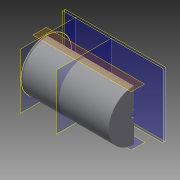
# Autodesk Inventor part: v1.0L
Saved by Autodesk Inventor 2015 SP2 (Build 190223200, 223)
## iProperties
Created: 2015-12-28
Part Number: v1.0L
Material: Ogólny
Document SubType Name: Modeling
Designer: amadi_000
Density: 1 g/cm^3
Appearance: Domyślna
Author: amadi_000
Autodesk Inventor part; units mm, degrees
ref_plane "YZ Plane" through (0, 0, 0) normal (1, 0, 0) x (0, 1, 0)
ref_plane "XZ Plane" through (0, 0, 0) normal (0, 1, 0) x (-1, 0, 0)
ref_plane "XY Plane" through (0, 0, 0) normal (0, 0, 1) x (1, 0, 0)
sketch "Szkic1" plane through (0, 0, 0) normal (1, 0, 0) x (0, 1, 0)
  circle A0 centre (0, 0) radius 42
  dimension "d0" = 84
  constraints: 1 centre point, 1 coincident
  measures "d0" diameter of A0
extrude "Wyciągnięcie proste1" add sketch "Szkic1" along normal blind 146
ref_plane "Płaszczyzna konstrukcyjna1" through (3, 0, 0) normal (-1, 0, 0) x (0, 0, 1)
sketch "Szkic2" plane through (3, 0, 0) normal (-1, 0, 0) x (0, 0, 1)
  point P0 (0, 0)
sketch "Szkic3" plane through (3, 0, 0) normal (-1, 0, 0) x (0, 0, 1)
  circle A0 centre (0, 0) radius 17
  circle A1 centre (0, 0) radius 15
  arc A2 (-17.4356, 36) -> (17.4356, 36) centre (0, 0) ccw
  line L0 (17.4356, 36) -> (-17.4356, 36)
  dimension "d4" = 34
  dimension "d5" = 30
  dimension "d10" = 80
  constraints: 3 centre point, 3 coincident, 2 end point, 2 point on circle, 1 horizontal
  measures "d4" diameter of A0
  measures "d5" diameter of A1
  measures "d10" diameter of A2
sketch "Szkic4" plane through (0, 0, 0) normal (-1, 0, 0) x (0, 0, 1)
  circle A0 centre (0, 0) radius 42 projected
  circle A1 centre (0, 0) radius 4.5
  circle A2 centre (10, 0) radius 2
  circle A3 centre (-10, 0) radius 2
  dimension "d6" = 9
  constraints: 3 centre point, 1 coincident
  measures "d6" diameter of A1
extrude "Wyciągnięcie proste2" cut sketch "Szkic4" against normal blind 146 contours A1 | A2 | A3
extrude "Wyciągnięcie proste3" cut sketch "Szkic3" against normal blind 140
ref_plane "Płaszczyzna konstrukcyjna2" through (63, 0, 0) normal (-1, 0, 0) x (0, 0, 1)
sketch "Szkic6" plane through (63, 0, 0) normal (-1, 0, 0) x (0, 0, 1)
  circle A0 centre (0, 0) radius 17
  constraints: 1 centre point, 1 coincident
extrude "Wyciągnięcie proste4" cut sketch "Szkic6" against normal blind 20
sketch "Szkic7" plane through (0, 0, 0) normal (-1, 0, 0) x (0, 0, 1)
  circle A0 centre (-10, 0) radius 2 projected
  circle A1 centre (10, 0) radius 2 projected
  circle A2 centre (0, 0) radius 4.5 projected
  circle A3 centre (0, 0) radius 42 projected
  point P0 (42, 0)
  constraints: 1 horizontal alignment, 1 other
ref_plane "Płaszczyzna konstrukcyjna3" through (0, 0, 42) normal (0, 0, 1) x (1, 0, 0)
sketch "Szkic8" plane through (0, 0, 42) normal (0, 0, 1) x (1, 0, 0)
  line L0 (0, -4.5) -> (0, 4.5) projected
  line L1 (146, 3) -> (0, 3)
  line L2 (0, 3) -> (0, -3)
  line L3 (0, -3) -> (146, -3)
  line L4 (146, -3) -> (146, 3)
  line L5 (146, 3) -> (0, -3) construction
  line L6 (0, 3) -> (146, -3) construction
  point P0 (0, 0)
  point P1 (73, 0)
  dimension "d16" = 6
  constraints: 12 end point, 2 midpoint, 2 parallel, 1 horizontal, 1 perpendicular, 1 point on line
  measures "d16" distance of L2.end L1.end
extrude "Wyciągnięcie proste5" add sketch "Szkic8" against normal blind 10
sketch "Szkic9" plane through (0, 0, 0) normal (-1, 0, 0) x (0, 0, 1)
  line L0 (42, 3) -> (42, -3) projected
  line L1 (42, 3) -> (41.8927, 3) projected
  arc A0 (41.8927, 3) -> (41.8927, -3) centre (0, 0) ccw projected
  line L2 (42, -3) -> (41.8927, -3) projected
  circle A1 centre (0, 0) radius 4.5 projected
  circle A2 centre (10, 0) radius 2 projected
  circle A3 centre (-10, 0) radius 2 projected
  point P0 (-42, 0)
  constraints: 1 point on circle
ref_plane "Płaszczyzna konstrukcyjna4" through (0, 0, -42) normal (0, 0, -1) x (-1, 0, 0)
sketch "Szkic10" plane through (0, 0, -42) normal (0, 0, -1) x (-1, 0, 0)
  line L0 (-146, -3) -> (0, -3)
  line L1 (0, -3) -> (0, 3)
  line L2 (0, 3) -> (-146, 3)
  line L3 (-146, 3) -> (-146, -3)
  line L4 (-146, -3) -> (0, 3) construction
  line L5 (0, -3) -> (-146, 3) construction
  point P0 (0, 0)
  point P1 (-73, 0)
  constraints: 12 end point, 2 midpoint, 2 parallel, 1 horizontal, 1 perpendicular
extrude "Wyciągnięcie proste6" add sketch "Szkic10" against normal blind 10
sketch "Szkic11" plane through (0, 0, 0) normal (-1, 0, 0) x (0, 0, 1)
  circle A0 centre (-10, 0) radius 2 projected
  circle A1 centre (10, 0) radius 2 projected
  circle A2 centre (0, 0) radius 4.5 projected
  line L0 (-42, -3) -> (-42, 3) projected
  line L1 (-42, -3) -> (-41.8927, -3) projected
  arc A3 (-41.8927, -3) -> (41.8927, -3) centre (0, 0) ccw projected
  line L2 (42, -3) -> (41.8927, -3) projected
  line L3 (42, 3) -> (42, -3) projected
  line L4 (42, 3) -> (41.8927, 3) projected
  arc A4 (41.8927, 3) -> (-41.8927, 3) centre (0, 0) ccw projected
  line L5 (-42, 3) -> (-41.8927, 3) projected
  arc A5 (41.8927, 3) -> (-41.8927, 3) centre (0, 0) ccw projected
  point P0 (0, 42)
  constraints: 2 point on circle
ref_plane "Płaszczyzna konstrukcyjna5" through (0, 42, 0) normal (0, 1, 0) x (-1, 0, 0)
sketch "Szkic12" plane through (0, 42, 0) normal (0, 1, 0) x (-1, 0, 0)
  circle A0 centre (-73, -36) radius 1
  circle A1 centre (-133, -36) radius 1
  circle A2 centre (-13, -36) radius 1
  circle A3 centre (-13, 36) radius 1
  circle A4 centre (-73, 36) radius 1
  circle A5 centre (-133, 36) radius 1
  point P0 (0, 0)
  constraints: 6 centre point
extrude "Wyciągnięcie proste7" cut sketch "Szkic12" against normal blind 45
ref_plane "Płaszczyzna konstrukcyjna7" through (0, 38, 0) normal (0, 1, 0) x (-1, 0, 0)
sketch "Szkic16" plane through (0, 42, 0) normal (0, 1, 0) x (-1, 0, 0)
  line L0 (-110, -6) -> (-36, -6)
  line L1 (-36, -6) -> (-36, 1)
  line L2 (-42, 6) -> (-104, 6)
  line L3 (-110, 1) -> (-110, -6)
  line L4 (-110, -6) -> (-36, 6) construction
  line L5 (-36, -6) -> (-110, 6) construction
  line L6 (-2, -15) -> (-144, -15)
  line L7 (-144, -15) -> (-144, 15)
  line L8 (-144, 15) -> (-2, 15)
  line L9 (-2, 15) -> (-2, -15)
  line L10 (-2, -15) -> (-144, 15) construction
  line L11 (-144, -15) -> (-2, 15) construction
  line L12 (-110, 1) -> (-104, 1)
  line L13 (-104, 1) -> (-104, 6)
  line L14 (-36, 1) -> (-42, 1)
  line L15 (-42, 1) -> (-42, 6)
  point P0 (0, 0)
  point P1 (-73, 0)
  dimension "d36" = 74
  dimension "d37" = 12
  constraints: 32 end point, 4 horizontal, 4 midpoint, 4 parallel, 4 perpendicular
  measures "d36" distance of L5.end L4.end
  measures "d37" distance of L4.end L0.end
extrude "Wyciągnięcie proste11" cut sketch "Szkic16" against normal blind 4.25 contours L3 L12 L13 L2 L15 L14 L1 L0
sketch "Szkic17" plane through (0, 38, 0) normal (0, 1, 0) x (-1, 0, 0)
  line L0 (-110.5, -6.5) -> (-35.5, -6.5)
  line L1 (-35.5, -6.5) -> (-35.5, 6.5)
  line L2 (-35.5, 6.5) -> (-110.5, 6.5)
  line L3 (-110.5, 6.5) -> (-110.5, -6.5)
  line L4 (-110.5, -6.5) -> (-35.5, 6.5) construction
  line L5 (-35.5, -6.5) -> (-110.5, 6.5) construction
  point P0 (0, 0)
  point P1 (-73, 0)
  dimension "d40" = 75
  dimension "d41" = 13
  constraints: 12 end point, 2 midpoint, 2 parallel, 1 horizontal, 1 perpendicular
  measures "d40" distance of L2.end L1.end
  measures "d41" distance of L1.end L0.end
extrude "Wyciągnięcie proste12" cut sketch "Szkic17" along normal blind 0.5
sketch "Szkic18" plane through (0, 0, 0) normal (-1, 0, 0) x (0, 0, 1)
  line L0 (42, 3) -> (42, -3) projected
  line L1 (42, 0) -> (-42, 0)
  line L2 (-42, 0) -> (-42, 42)
  line L3 (-42, 42) -> (42, 42)
  line L4 (42, 42) -> (42, 0)
  constraints: 8 end point, 2 parallel, 1 horizontal, 1 midpoint, 1 perpendicular
extrude "Wyciągnięcie proste13" cut sketch "Szkic18" against normal blind 146
